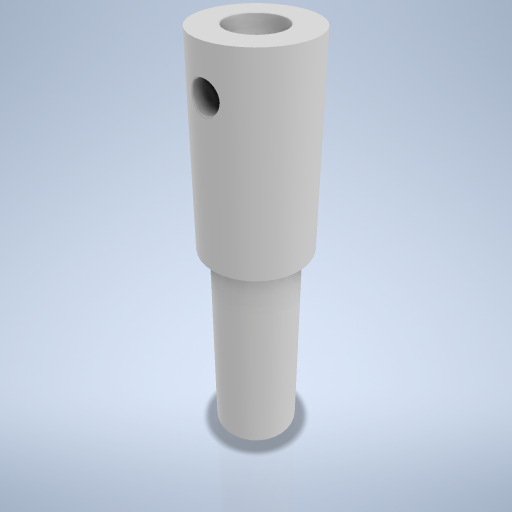
# Autodesk Inventor part: 19
Saved by Autodesk Inventor 2024.2 (Build 282272000, 272)
## iProperties
Created: 2024-05-05
Part Number: 19
Material: Generisch
Document SubType Name: Modeling
Designer: Fabri
Density: 1 g/cm^3
Appearance: Vorgabe
Author: Fabri
Autodesk Inventor part; units mm, degrees
ref_plane "YZ Plane" through (0, 0, 0) normal (1, 0, 0) x (0, 1, 0)
ref_plane "XY Plane" through (0, 0, 0) normal (0, 0, 1) x (1, 0, 0)
sketch "Skizze1" plane through (0, 0, 0) normal (0, 1, 0) x (-1, 0, 0)
  line L0 (0, 0) -> (18, 0)
  line L1 (18, 0) -> (18, -5)
  line L2 (18, -5) -> (18, -5)
  line L3 (18, -5) -> (18, -11)
  line L4 (18, -11) -> (18, -11)
  line L5 (18, -11) -> (18, -66)
  line L6 (18, -66) -> (14, -66)
  line L7 (14, -66) -> (14, -140)
  line L8 (14, -140) -> (0, -140)
  line L9 (0, -140) -> (0, 0)
  point P0 (18, -8)
  dimension "d0" = 74
  dimension "d1" = 66
  dimension "d5" = 36
  dimension "d6" = 28
  constraints: 20 end point, 8 perpendicular, 2 horizontal, 1 coincident, 1 midpoint, 1 vertical alignment
  measures "d0" distance between parallel lines of L8 L6
  measures "d1" distance between parallel lines of L0 L6
  measures "d5" diameter of L5 L9
  measures "d6" diameter of L7 L9
revolve "Umdrehung1" add sketch "Skizze1" angle 360 about axis through (0, 0, -140) along (0, 0, 1)
ref_plane "Arbeitsebene1" through (0, 18, 0) normal (0, 1, 0) x (-1, 0, 0)
sketch "Skizze2" plane through (0, 18, 0) normal (0, 1, 0) x (-1, 0, 0)
  point P0 (0, 0)
  point P1 (0, -14)
  dimension "d9" = 14
  constraints: 1 vertical alignment
  measures "d9" distance of point (0, 0) point (0, -14)
hole "Bohrung1" at (0, 18, -14) direction (0, -1, 0) diameter 10 end through all
sketch "Skizze3" plane through (0, 0, 0) normal (0, 0, 1) x (1, 0, 0)
  circle A0 centre (0, 0) radius 9
  dimension "d17" = 18
  constraints: 1 centre point, 1 coincident
  measures "d17" diameter of A0
extrude "Extrusion1" cut sketch "Skizze3" against normal blind 90
chamfer "Fasen1" distance 2 angle 45 1 edges at (14, 0, -140)
